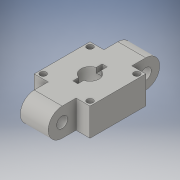
# Autodesk Inventor part: bottom_anchor_v3
Saved by Autodesk Inventor 2016 (Build 200138000, 138)
## iProperties
Created: 2016-02-24
Part Number: bottom_anchor_v3
Material: Generic
Document SubType Name: Modeling
Designer: Matt Ruffner
Density: 1 g/cm^3
Appearance: Default
Author: Matt Ruffner
Autodesk Inventor part; units mm, degrees
ref_plane "YZ Plane" through (0, 0, 0) normal (1, 0, 0) x (0, 1, 0)
ref_plane "XZ Plane" through (0, 0, 0) normal (0, 1, 0) x (-1, 0, 0)
ref_plane "XY Plane" through (0, 0, 0) normal (0, 0, 1) x (1, 0, 0)
sketch "Sketch1" plane through (0, 0, 0) normal (0, 1, 0) x (-1, 0, 0)
  line L0 (8.9115, 17.7017) -> (-16.4885, 17.7017)
  line L1 (-16.4885, 17.7017) -> (-16.4885, -33.0983)
  line L2 (-16.4885, -33.0983) -> (8.9115, -33.0983)
  line L3 (8.9115, -33.0983) -> (8.9115, 17.7017)
  line L4 (8.9115, 17.7017) -> (2.5615, 17.7017)
  line L5 (2.5615, 17.7017) -> (2.5615, 5.0017)
  line L6 (2.5615, 5.0017) -> (8.9115, 5.0017)
  line L7 (8.9115, 5.0017) -> (8.9115, 17.7017)
  line L8 (-16.4885, 17.7017) -> (-10.1385, 17.7017)
  line L9 (-10.1385, 17.7017) -> (-10.1385, 5.0017)
  line L10 (-10.1385, 5.0017) -> (-16.4885, 5.0017)
  line L11 (-16.4885, 5.0017) -> (-16.4885, 17.7017)
  line L12 (8.9115, -33.0983) -> (2.5615, -33.0983)
  line L13 (2.5615, -33.0983) -> (2.5615, -20.3983)
  line L14 (2.5615, -20.3983) -> (8.9115, -20.3983)
  line L15 (8.9115, -20.3983) -> (8.9115, -33.0983)
  line L16 (-16.4885, -33.0983) -> (-10.1385, -33.0983)
  line L17 (-10.1385, -33.0983) -> (-10.1385, -20.3983)
  line L18 (-10.1385, -20.3983) -> (-16.4885, -20.3983)
  line L19 (-16.4885, -20.3983) -> (-16.4885, -33.0983)
  circle A0 centre (-3.7885, -7.6983) radius 4.1275
  point P0 (0, 0)
  dimension "d0" = 25.4
  dimension "d1" = 50.8
  dimension "d2" = 6.35
  dimension "d3" = 12.7
  dimension "d4" = 6.35
  dimension "d5" = 12.7
  dimension "d6" = 6.35
  dimension "d7" = 12.7
  dimension "d8" = 6.35
  dimension "d9" = 12.7
  dimension "d10" = 8.255
  constraints: 40 end point, 10 parallel, 5 horizontal, 5 perpendicular, 1 centre point
  measures "d0" distance of L2.end L1.end
  measures "d1" distance of L1.end L0.end
  measures "d2" distance of L6.end L5.end
  measures "d3" distance of L5.end L4.end
  measures "d4" distance of L9.end L10.end
  measures "d5" distance of L8.end L9.end
  measures "d6" distance of L13.end L14.end
  measures "d7" distance of L12.end L13.end
  measures "d8" distance of L18.end L17.end
  measures "d9" distance of L17.end L16.end
  measures "d10" diameter of A0
extrude "Extrusion1" add sketch "Sketch1" against normal blind 12.7 contours L5 L6 L3 L14 L13 L2 L17 L18 L1 L10 L9 L0
sketch "Sketch2" plane through (10.1385, -12.7, 17.7017) normal (1, 0, 0) x (0, 0, -1)
  circle A0 centre (6.35, 6.35) radius 2.5083
  line L0 (0, 0) -> (0, 12.7) projected
  line L1 (12.7, 0) -> (0, 0) projected
  circle A1 centre (44.45, 6.35) radius 2.5083
  line L2 (38.1, 12.7) -> (50.8, 12.7) projected
  line L3 (50.8, 12.7) -> (50.8, 0) projected
  point P0 (17.7017, 12.7)
  dimension "d13" = 5.0165
  dimension "d14" = 6.35
  dimension "d15" = 6.35
  dimension "d16" = 5.0165
  dimension "d17" = 6.35
  dimension "d18" = 6.35
  constraints: 2 centre point
  measures "d13" diameter of A0
  measures "d14" distance from line of L0 A0.centre
  measures "d15" distance from line of L1 A0.centre
  measures "d16" diameter of A1
  measures "d17" distance from line of L2 A1.centre
  measures "d18" distance from line of L3 A1.centre
extrude "Extrusion2" cut sketch "Sketch2" against normal blind 12.7
fillet "Fillet1" radius 6.35 4 edges at (3.7885, 0, 17.7017) (3.7885, -12.7, 17.7017) (3.7885, 0, -33.0983) (3.7885, -12.7, -33.0983)
sketch "Sketch3" plane through (0, 0, 0) normal (0, 1, 0) x (1, 0, 0)
  circle A0 centre (-6.8795, -2.9697) radius 1.397
  line L0 (-8.9115, -5.0017) -> (-2.5615, -5.0017) projected
  line L1 (-8.9115, 20.3983) -> (-8.9115, -5.0017) projected
  circle A1 centre (14.4565, -2.9697) radius 1.397
  line L2 (16.4885, -5.0017) -> (16.4885, 20.3983) projected
  circle A2 centre (14.4565, 18.3663) radius 1.397
  line L3 (16.4885, 20.3983) -> (10.1385, 20.3983) projected
  circle A3 centre (-6.8795, 18.3663) radius 1.397
  point P0 (0, 0)
  dimension "d22" = 2.794
  dimension "d23" = 2.032
  dimension "d24" = 2.032
  dimension "d25" = 2.794
  dimension "d26" = 2.032
  dimension "d27" = 2.794
  dimension "d28" = 2.032
  dimension "d29" = 2.794
  constraints: 4 centre point
  measures "d22" diameter of A0
  measures "d23" distance from line of L0 A0.centre
  measures "d24" distance from line of L1 A0.centre
  measures "d25" diameter of A1
  measures "d26" distance from line of L2 A1.centre
  measures "d27" diameter of A2
  measures "d28" distance from line of L3 A2.centre
  measures "d29" diameter of A3
extrude "Extrusion3" cut sketch "Sketch3" against normal blind 7.62
sketch "Sketch4" plane through (0, 0, 0) normal (0, 1, 0) x (1, 0, 0)
  line L0 (2.6455, 1.0308) -> (4.9315, 1.0308)
  line L1 (4.9315, 1.0308) -> (4.9315, 3.7322)
  line L2 (2.6455, 3.7322) -> (2.6455, 1.0308)
  circle A0 centre (3.7885, 7.6983) radius 4.1275 projected
  line L3 (4.9315, 14.3658) -> (2.6455, 14.3658)
  line L4 (2.6455, 14.3658) -> (2.6455, 11.6644)
  line L5 (4.9315, 11.6644) -> (4.9315, 14.3658)
  point P0 (0, 0)
  dimension "d32" = 2.286
  dimension "d34" = 8.255
  dimension "d36" = 1.143
  dimension "d37" = 2.286
  constraints: 12 end point, 4 point on circle, 2 parallel, 2 perpendicular
  measures "d32" distance of L0.start L0.end
  measures "d34" diameter of A0
  measures "d36" distance from line of A0.centre L1
  measures "d37" distance of L5.end L4.start
extrude "Extrusion4" cut sketch "Sketch4" against normal blind 2.286 contours L2 A0 L1 L0 | L4 L3 L5 A0
body "Solid1"
